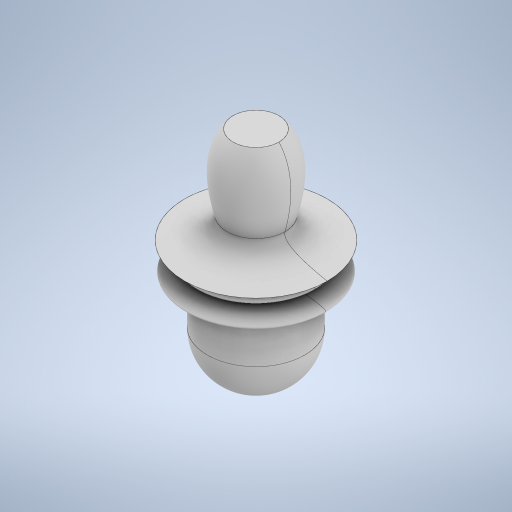
# Autodesk Inventor part: Joystick upper
Saved by Autodesk Inventor 2023 (Build 270158000, 158)
## iProperties
Created: 2023-11-15
Part Number: Joystick upper
Material: Generic
Document SubType Name: Modeling
Designer: DELL
Density: 1 g/cm^3
Appearance: Default
Author: DELL
Autodesk Inventor part; units mm, degrees
ref_plane "YZ Plane" through (0, 0, 0) normal (1, 0, 0) x (0, 1, 0)
ref_plane "XZ Plane" through (0, 0, 0) normal (0, 1, 0) x (-1, 0, 0)
ref_plane "XY Plane" through (0, 0, 0) normal (0, 0, 1) x (1, 0, 0)
sketch "Sketch1" plane through (0, 0, 0) normal (0, 0, 1) x (1, 0, 0)
  line L0 (0, 0) -> (17, 0)
  line L1 (17, 0) -> (17, 15)
  line L2 (17, 15) -> (32.9081, 17.0364) construction
  line L3 (32.9081, 17.0364) -> (14.4853, 18.8023) construction
  spline S0 degree 2 poles (17, 15) (32.9081, 17.0364) (14.4853, 18.8023) knots 1 1 1 2 2 2
  line L4 (14.4853, 18.8023) -> (7.0733, 19.5128) construction
  line L5 (7.0733, 19.5128) -> (21.952, 20.7075) construction
  line L6 (21.952, 20.7075) -> (26.5373, 22.3819) construction
  line L7 (26.5373, 22.3819) -> (13.5554, 23.0501) construction
  spline S1 degree 4 poles (14.4853, 18.8023) (7.0733, 19.5128) (21.952, 20.7075) (26.5373, 22.3819) (13.5554, 23.0501) knots 1 1 1 1 1 2 2 2 2 2
  line L8 (13.5554, 23.0501) -> (13.5554, 26.2794)
  line L9 (13.5554, 23.0501) -> (16.7847, 23.0501) construction
  line L10 (13.5554, 26.2794) -> (24.8704, 26.2794)
  line L11 (24.8704, 26.2794) -> (8.7793, 29.4014) construction
  line L12 (8.7793, 29.4014) -> (10.1424, 33.878) construction
  spline S2 degree 2 poles (24.8704, 26.2794) (8.7793, 29.4014) (10.1424, 33.878) knots 1 1 1 2 2 2
  line L13 (10.1424, 33.878) -> (15.0402, 51.9555) construction
  line L14 (15.0402, 51.9555) -> (8, 59.878) construction
  spline S3 degree 2 poles (10.1424, 33.878) (15.0402, 51.9555) (8, 59.878) knots 1 1 1 2 2 2
  line L15 (8, 59.878) -> (0, 59.878)
  line L16 (8, 59.878) -> (16, 59.878) construction
  line L17 (0, 59.878) -> (0, 0)
  arc A0 (0, -4.7625) -> (17, 15) centre (6.8127, 6.5702) ccw
  point P0 (9.4608, 31.6397)
  dimension "d0" = 17
  dimension "d1" = 15
  dimension "d3" = 11.315
  dimension "d5" = 59.878
  dimension "d6" = 3.2294
  dimension "d7" = 8
  dimension "d8" = 26
  dimension "d9" = 4.2477
  dimension "d10" = 3.8024
  dimension "d13" = 9.4608
  dimension "d14" = 10.1424
  constraints: 16 end point, 3 horizontal, 3 perpendicular, 2 equal length, 2 point on circle, 1 centre point, 1 midpoint, 12 other
  measures "d0" distance of L0.start L0.end
  measures "d1" distance of L0.end L1.end
  measures "d3" distance of L8.end L10.end
  measures "d5" distance of L15.end L0.start
  measures "d6" distance of L7.end L8.end
  measures "d7" distance of L14.end L15.end
  measures "d8" distance from line of L16 L12.end
  measures "d9" vertical distance of L3.end L7.end
  measures "d10" vertical distance of L3.end L1.end
  measures "d13" distance from line of L17 point (9.461, 31.64)
  measures "d14" distance from line of L17 L12.end
revolve "Revolution1" add sketch "Sketch1" angle 360 about axis through (0, 59.878, 0) along (0, -1, 0)
sketch "Sketch2" plane through (0, 0, 0) normal (0, 0, 1) x (1, 0, 0)
  line L0 (17, 15) -> (17, 0) projected
  line L1 (-17, 0) -> (17, 0) projected
  arc A0 (0, -17) -> (17, 0) centre (0, 0) ccw
  line L2 (0, -17) -> (0, 0)
  constraints: 2 end point, 2 point on circle, 1 centre point, 1 coincident, 1 perpendicular
revolve "Revolution2" add sketch "Sketch2" angle 360 about axis through (0, -17, 0) along (0, 1, 0)
body "Solid1"
